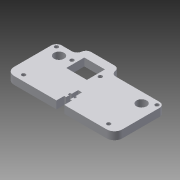
# Autodesk Inventor part: XcrLeft_b
Saved by Autodesk Inventor 2013 (Build 170138000, 138)
## iProperties
Created: 2015-01-14
Part Number: XcrLeft_b
Material: Generic
Document SubType Name: Modeling
Designer: dzban
Density: 1 g/cm^3
Author: dzban
Autodesk Inventor part; units mm, degrees
ref_plane "YZ Plane" through (0, 0, 0) normal (1, 0, 0) x (0, 1, 0)
ref_plane "XZ Plane" through (0, 0, 0) normal (0, 1, 0) x (-1, 0, 0)
ref_plane "XY Plane" through (0, 0, 0) normal (0, 0, 1) x (1, 0, 0)
sketch "Sketch1" plane through (0, 0, 0) normal (0, 0, 1) x (1, 0, 0)
  arc A0 (-84, -33) -> (-78, -39) centre (-78, -33) ccw
  line L0 (-78, -39) -> (-45, -39)
  line L1 (-45, -39) -> (-45, -33)
  line L2 (-45, -33) -> (-43.5, -33)
  line L3 (-43.5, -33) -> (-43.5, -30.5)
  line L4 (-43.5, -30.5) -> (-44.75, -30.5)
  line L5 (-44.75, -30.5) -> (-44.75, -28.7)
  line L6 (-44.75, -28.7) -> (-43.5, -28.7)
  line L7 (-43.5, -28.7) -> (-43.5, -23.7)
  line L8 (-43.5, -23.7) -> (-40.5, -23.7)
  line L9 (-40.5, -23.7) -> (-40.5, -28.7)
  line L10 (-40.5, -28.7) -> (-39.25, -28.7)
  line L11 (-39.25, -28.7) -> (-39.25, -30.5)
  line L12 (-39.25, -30.5) -> (-40.5, -30.5)
  line L13 (-40.5, -30.5) -> (-40.5, -33)
  line L14 (-40.5, -33) -> (-39, -33)
  line L15 (-39, -33) -> (-39, -39)
  line L16 (-39, -39) -> (-6, -39)
  arc A1 (-6, -39) -> (0, -33) centre (-6, -33) ccw
  line L17 (0, -33) -> (0, -4)
  arc A2 (0, -4) -> (-4, 0) centre (-4, -4) ccw
  line L18 (-4, 0) -> (-38, 0)
  arc A3 (-41.9686, 3.5) -> (-38, 0) centre (-38, 4) ccw
  arc A4 (-41.9686, 3.5) -> (-45.9373, 7) centre (-45.9373, 3) ccw
  line L19 (-45.9373, 7) -> (-64.0627, 7)
  arc A5 (-64.0627, 7) -> (-68.0314, 3.5) centre (-64.0627, 3) ccw
  arc A6 (-72, 0) -> (-68.0314, 3.5) centre (-72, 4) ccw
  line L20 (-72, 0) -> (-80, 0)
  arc A7 (-80, 0) -> (-84, -4) centre (-80, -4) ccw
  line L21 (-84, -4) -> (-84, -33)
  line L22 (-63, 0.6) -> (-47, 0.6)
  line L23 (-47, 0.6) -> (-47, -13.4)
  line L24 (-47, -13.4) -> (-63, -13.4)
  line L25 (-63, -13.4) -> (-63, 0.6)
  circle A8 centre (-81, -3) radius 1.5
  circle A9 centre (-9, -34.5) radius 1.5
  circle A10 centre (-3, -3) radius 1.5
  circle A11 centre (-66, -6) radius 1.5
  circle A12 centre (-44, -6) radius 1.5
  circle A13 centre (-75, -34.5) radius 1.5
  circle A14 centre (-10, -8) radius 3.94
  circle A15 centre (-74, -8) radius 3.94
  point P0 (0, 0)
  constraints: 52 end point, 16 centre point, 16 point on circle
extrude "Extrusion1" add sketch "Sketch1" along normal blind 6
body "Solid1"
